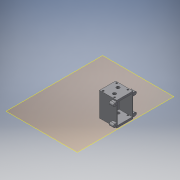
# Autodesk Inventor part: shifter box 1
Saved by Autodesk Inventor 2017 (Build 210142000, 142)
## iProperties
Created: 2018-04-17
Part Number: shifter box 1
Material: Generic
Document SubType Name: Modeling
Designer: RKL
Density: 1 g/cm^3
Appearance: Default
Mass: 39.3602 g
Surface Area: 235.41 cm^2
Volume: 39.3602 cm^3
Author: RKL
Autodesk Inventor part; units mm, degrees
ref_plane "YZ Plane" through (0, 0, 0) normal (1, 0, 0) x (0, 1, 0)
ref_plane "XZ Plane" through (0, 0, 0) normal (0, 1, 0) x (-1, 0, 0)
ref_plane "XY Plane" through (0, 0, 0) normal (0, 0, 1) x (1, 0, 0)
ref_plane "Work Plane1" through (0, 0, 0) normal (0, 0, 1) x (1, 0, 0)
sketch "Sketch1" plane through (0, 0, 0) normal (0, 0, 1) x (1, 0, 0)
  circle A0 centre (55.8916, -14.7421) radius 1.397 construction
  circle A1 centre (83.8916, 18.2579) radius 1.397 construction
  circle A2 centre (83.8916, -14.7421) radius 1.397 construction
  circle A3 centre (55.8916, 18.2579) radius 1.397 construction
  circle A4 centre (-68.9014, -27.1927) radius 1.905 construction
  circle A5 centre (69.9706, -24.3098) radius 1.905 construction
  arc A6 (-6.1836, 105.2542) -> (-60.0665, 55.7083) centre (-0.9442, 45.4834) ccw construction
  arc A7 (-60.0665, 55.7083) -> (-61.034, 47.7681) centre (-60.6164, 51.7463) ccw construction
  line L0 (-61.034, 47.7681) -> (-68.4839, -23.2145) construction
  arc A8 (-68.4839, -23.2145) -> (-69.2051, -31.1811) centre (-68.9014, -27.1927) ccw construction
  arc A9 (-69.2051, -31.1811) -> (-1.8309, -104.453) centre (0.7162, -34.4994) ccw construction
  arc A10 (-1.8309, -104.453) -> (6.1641, -104.2871) centre (2.169, -104.4843) ccw construction
  arc A11 (6.1641, -104.2871) -> (70.4395, -28.2823) centre (0.7162, -34.4994) ccw construction
  arc A12 (70.4395, -28.2823) -> (69.3883, -20.3524) centre (69.9706, -24.3098) ccw construction
  line L1 (69.3883, -20.3524) -> (69.0778, -18.2421) construction
  line L2 (87.8916, -18.2421) -> (69.0778, -18.2421) construction
  line L3 (87.8916, 21.7579) -> (87.8916, -18.2421) construction
  line L4 (63.1925, 21.7579) -> (87.8916, 21.7579) construction
  line L5 (63.1925, 21.7579) -> (58.999, 50.2599) construction
  arc A13 (58.999, 50.2599) -> (57.7029, 58.1531) centre (58.4167, 54.2173) ccw construction
  arc A14 (57.7029, 58.1531) -> (1.8102, 105.4201) centre (-0.9442, 45.4834) ccw construction
  arc A15 (1.8102, 105.4201) -> (-6.1836, 105.2542) centre (-2.1895, 105.4705) ccw construction
  circle A16 centre (58.4167, 54.2173) radius 1.905 construction
  circle A17 centre (-2.1895, 105.4705) radius 1.905 construction
  circle A18 centre (-60.6164, 51.7463) radius 1.905 construction
  circle A19 centre (2.169, -104.4843) radius 1.905 construction
  circle A20 centre (-0.9442, 45.4834) radius 6.75 construction
  circle A21 centre (75.8916, -7.1378) radius 4 projected
  circle A22 centre (66.7556, 10.6536) radius 4 projected
  line L6 (87.8916, -18.2421) -> (87.8916, 21.7579)
  line L7 (87.8916, 21.7579) -> (49.8916, 21.7579)
  line L8 (49.8916, 21.7579) -> (49.8916, -18.2421)
  line L9 (49.8916, -18.2421) -> (87.8916, -18.2421)
  circle A23 centre (83.8916, -14.7421) radius 1.905
  circle A24 centre (55.8916, -14.7421) radius 1.905
  circle A25 centre (55.8916, 18.2579) radius 1.905
  circle A26 centre (83.8916, 18.2579) radius 1.905
  point P0 (0, 0)
  dimension "d0" = 3.81
  dimension "d1" = 38
  constraints: 8 end point, 4 centre point, 4 coincident, 3 equal length, 3 equal radius, 1 perpendicular
  measures "d0" diameter of A23
  measures "d1" distance between parallel lines of L3 L8
extrude "Extrusion1" add sketch "Sketch1" along normal blind 5
sketch "Sketch2" plane through (0, 0, 5) normal (0, 0, 1) x (1, 0, 0)
  circle A0 centre (66.7556, 10.6536) radius 4 construction
  circle A1 centre (75.8916, -7.1378) radius 4 construction
  circle A2 centre (83.8916, 18.2579) radius 1.905 construction
  circle A3 centre (55.8916, 18.2579) radius 1.905 construction
  circle A4 centre (55.8916, -14.7421) radius 1.905 construction
  circle A5 centre (83.8916, -14.7421) radius 1.905 construction
  line L0 (87.8916, -18.2421) -> (87.8916, 21.7579) construction
  line L1 (87.8916, 21.7579) -> (49.8916, 21.7579) construction
  line L2 (49.8916, 21.7579) -> (49.8916, -18.2421) construction
  line L3 (49.8916, -18.2421) -> (87.8916, -18.2421) construction
  line L4 (87.8916, -18.2421) -> (49.8916, -18.2421)
  line L5 (49.8916, -18.2421) -> (49.8916, -16.6471)
  line L6 (49.8916, -16.6471) -> (87.8916, -16.6471)
  line L7 (87.8916, -16.6471) -> (87.8916, -18.2421)
  line L8 (87.8916, 21.7579) -> (49.8916, 21.7579) projected
  line L9 (87.8916, 21.7579) -> (49.8916, 21.7579)
  line L10 (49.8916, 21.7579) -> (49.8916, 20.1629)
  line L11 (49.8916, 20.1629) -> (87.8916, 20.1629)
  line L12 (87.8916, 20.1629) -> (87.8916, 21.7579)
  line L13 (49.8916, -16.6471) -> (53.9866, -16.6471)
  line L14 (53.9866, -16.6471) -> (53.9866, 20.1629)
  line L15 (53.9866, 20.1629) -> (49.8916, 20.1629)
  line L16 (49.8916, 20.1629) -> (49.8916, -16.6471)
  circle A6 centre (55.8916, -14.7421) radius 1.905 projected
  point P0 (0, 0)
  constraints: 24 end point, 6 parallel, 3 horizontal, 3 perpendicular, 3 point on line, 3 tangent
extrude "Extrusion2" add sketch "Sketch2" along normal blind 50 contours L4 L5 L6 L7 | L16 L11 L14 L6 | L10 L8 L12 L11
sketch "Sketch3" plane through (0, 0, 55) normal (0, 0, 1) x (1, 0, 0)
  line L0 (55.8916, -16.6471) -> (83.8916, -16.6471) projected
  circle A0 centre (83.8916, -14.7421) radius 1.905 projected
  line L1 (83.8916, -16.6471) -> (87.8916, -16.6471) projected
  line L2 (87.8916, -16.6471) -> (87.8916, 20.1629) projected
  line L3 (87.8916, 20.1629) -> (83.8916, 20.1629) projected
  circle A1 centre (83.8916, 18.2579) radius 1.905 projected
  line L4 (83.8916, 20.1629) -> (55.8916, 20.1629) projected
  arc A2 (53.9866, 18.2579) -> (55.8916, 20.1629) centre (55.8916, 18.2579) ccw projected
  line L5 (53.9866, 18.2579) -> (53.9866, -14.7421) projected
  arc A3 (55.8916, -16.6471) -> (53.9866, -14.7421) centre (55.8916, -14.7421) ccw projected
  circle A4 centre (66.7556, 10.6536) radius 4 projected
  circle A5 centre (75.8916, -7.1378) radius 4 projected
  line L6 (53.9866, 20.1629) -> (87.8916, 20.1629) projected
  line L7 (87.8916, 20.1629) -> (87.8916, 21.7579) projected
  line L8 (87.8916, 21.7579) -> (49.8916, 21.7579) projected
  line L9 (49.8916, 21.7579) -> (49.8916, -18.2421) projected
  line L10 (49.8916, -18.2421) -> (87.8916, -18.2421) projected
  line L11 (87.8916, -18.2421) -> (87.8916, -16.6471) projected
  line L12 (87.8916, -16.6471) -> (53.9866, -16.6471) projected
  line L13 (53.9866, -16.6471) -> (53.9866, 20.1629) projected
  point P0 (0, 0)
  constraints: 2 vertical alignment
extrude "Extrusion3" add sketch "Sketch3" along normal blind 5 contours A3 L5 A2 L4 L3 L2 L1 L0 | L0 L1 L11 L10 L9 L8 L7 L3 L4 L6 L13 L5 L12
sketch "Sketch4" plane through (87.8916, -18.2421, 0) normal (1, 0, 0) x (0, 0, -1)
  line L0 (-5, 38.405) -> (-55, 38.405) projected
  line L1 (-5, 1.595) -> (-5, 38.405) projected
  line L2 (-5, 1.595) -> (-55, 1.595) projected
  line L3 (-55, 1.595) -> (-55, 38.405) projected
  line L4 (0, 40) -> (-60, 40) projected
  line L5 (-60, 0) -> (-60, 40) projected
  line L6 (0, 0) -> (-60, 0) projected
  line L7 (0, 0) -> (0, 40) projected
  point P0 (0, 18.2421)
extrude "Extrusion4" add sketch "Sketch4" along normal blind 5
sketch "Sketch5" plane through (0, 0, 5) normal (0, 0, 1) x (1, 0, 0)
  line L0 (55.8916, -16.6471) -> (83.8916, -16.6471) projected
  circle A0 centre (83.8916, -14.7421) radius 1.905 projected
  line L1 (83.8916, -16.6471) -> (92.8916, -16.6471) projected
  line L2 (92.8916, 20.1629) -> (92.8916, -16.6471) projected
  line L3 (92.8916, 20.1629) -> (83.8916, 20.1629) projected
  circle A1 centre (83.8916, 18.2579) radius 1.905 projected
  line L4 (83.8916, 20.1629) -> (55.8916, 20.1629) projected
  arc A2 (53.9866, 18.2579) -> (55.8916, 20.1629) centre (55.8916, 18.2579) ccw projected
  line L5 (53.9866, 18.2579) -> (53.9866, -14.7421) projected
  arc A3 (55.8916, -16.6471) -> (53.9866, -14.7421) centre (55.8916, -14.7421) ccw projected
  circle A4 centre (66.7556, 10.6536) radius 4 projected
  circle A5 centre (75.8916, -7.1378) radius 4 projected
  line L6 (59.9866, 20.1629) -> (59.9866, 13.1536)
  line L7 (59.9866, 13.1536) -> (53.9866, 13.1536)
  line L8 (53.9866, 8.1536) -> (59.9866, 8.1536)
  line L9 (59.9866, 8.1536) -> (59.9866, -4.6378)
  line L10 (59.9866, -4.6378) -> (53.9866, -4.6378)
  line L11 (53.9866, -9.6378) -> (59.9866, -9.6378)
  line L12 (59.9866, -9.6378) -> (59.9866, -16.6471)
  line L13 (59.9866, -9.6378) -> (59.9866, -4.6378) construction
  line L14 (59.9866, 8.1536) -> (59.9866, 13.1536) construction
  point P0 (0, 0)
  point P1 (59.9866, -7.1378)
  point P2 (59.9866, 10.6536)
  dimension "d10" = 5
  dimension "d11" = 6
  dimension "d12" = 5
  constraints: 18 end point, 10 point on line, 3 perpendicular, 2 equal length, 2 horizontal alignment, 2 midpoint, 2 vertical, 2 vertical alignment
  measures "d10" distance of L11.end L9.end
  measures "d11" distance between parallel lines of L5 L12
  measures "d12" distance of L8.end L6.end
extrude "Extrusion5" add sketch "Sketch5" along normal up to next contours A3 L5 L11 L12 L0 | L5 L8 L9 L10 | L5 A2 L4 L6 L7
sketch "Sketch6" plane through (92.8916, -18.2421, 0) normal (1, 0, 0) x (0, 0, -1)
  line L0 (-5, 38.405) -> (-5, 1.595) construction
  line L1 (-5, 1.595) -> (-55, 1.595) construction
  line L2 (-55, 1.595) -> (-55, 38.405) construction
  line L3 (-55, 38.405) -> (-5, 38.405) construction
  line L4 (0, 40) -> (-60, 40) construction
  line L5 (-60, 40) -> (-60, 0) construction
  line L6 (-60, 0) -> (0, 0) construction
  line L7 (0, 0) -> (0, 40) construction
  line L8 (-60, 0) -> (0, 0) construction
  line L9 (-30, 0) -> (-30, 40) construction
  line L10 (-52.5, 45) -> (-7.5, 45) construction
  line L11 (-7.5, 45) -> (-7.5, -5) construction
  line L12 (-7.5, -5) -> (-52.5, -5) construction
  line L13 (-52.5, -5) -> (-52.5, 45) construction
  line L14 (-52.5, 45) -> (-7.5, -5) construction
  line L15 (-7.5, 45) -> (-52.5, -5) construction
  circle A0 centre (-7.5, -5) radius 1.397
  circle A1 centre (-52.5, -5) radius 1.397
  circle A2 centre (-7.5, 45) radius 1.397
  circle A3 centre (-52.5, 45) radius 1.397
  line L16 (-7.5, -5) -> (-7.5, 0) construction
  line L17 (-11.5, -5) -> (-11.5, 0)
  line L18 (-3.5, 0) -> (-3.5, -5)
  arc A4 (-11.5, -5) -> (-3.5, -5) centre (-7.5, -5) ccw
  arc A5 (-3.5, 0) -> (-11.5, 0) centre (-7.5, 0) ccw construction
  line L19 (-52.5, -5) -> (-52.5, 0) construction
  line L20 (-48.5, -5) -> (-48.5, 0)
  line L21 (-56.5, 0) -> (-56.5, -5)
  arc A6 (-56.5, -5) -> (-48.5, -5) centre (-52.5, -5) ccw
  arc A7 (-48.5, 0) -> (-56.5, 0) centre (-52.5, 0) ccw construction
  line L22 (-52.5, 45) -> (-52.5, 40) construction
  line L23 (-48.5, 45) -> (-48.5, 40)
  line L24 (-56.5, 40) -> (-56.5, 45)
  arc A8 (-48.5, 45) -> (-56.5, 45) centre (-52.5, 45) ccw
  arc A9 (-56.5, 40) -> (-48.5, 40) centre (-52.5, 40) ccw construction
  line L25 (-7.5, 45) -> (-7.5, 40) construction
  line L26 (-11.5, 45) -> (-11.5, 40)
  line L27 (-3.5, 40) -> (-3.5, 45)
  arc A10 (-3.5, 45) -> (-11.5, 45) centre (-7.5, 45) ccw
  arc A11 (-11.5, 40) -> (-3.5, 40) centre (-7.5, 40) ccw construction
  line L28 (-3.5, 0) -> (-11.5, 0)
  line L29 (-56.5, 0) -> (-48.5, 0)
  line L30 (-56.5, 40) -> (-48.5, 40)
  line L31 (0, 40) -> (-60, 40) projected
  line L32 (-11.5, 40) -> (-3.5, 40)
  point P0 (0, 18.2421)
  point P1 (-30, 20)
  point P2 (-7.5, -2.5)
  point P3 (-52.5, -2.5)
  point P4 (-52.5, 42.5)
  point P5 (-7.5, 42.5)
  dimension "d15" = 2.794
  dimension "d16" = 50
  dimension "d17" = 45
  dimension "d18" = 4
  constraints: 54 end point, 16 point on circle, 16 tangent, 12 centre point, 9 midpoint, 8 point on line, 6 equal radius, 6 parallel, 4 coincident, 3 collinear, 2 perpendicular, 1 horizontal
  measures "d15" diameter of A0
  measures "d16" distance of L12.end L10.start
  measures "d17" distance of L11.end L12.end
  measures "d18" radius of A4
extrude "Extrusion6" add sketch "Sketch6" against normal blind 10
body "Solid1"
